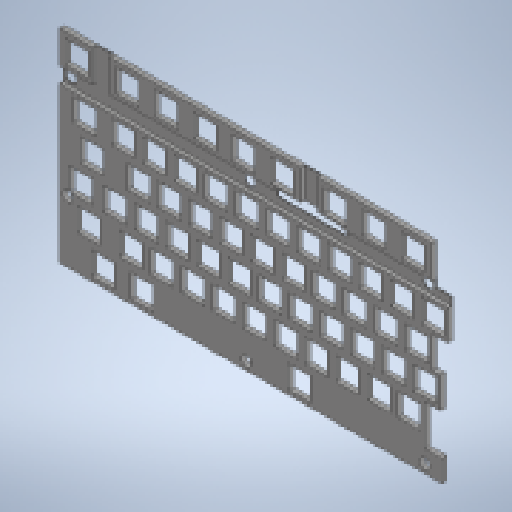
# Autodesk Inventor part: Left Plate
Saved by Autodesk Inventor 2025 (Build 290162000, 162)
## iProperties
Created: 2024-08-12
Part Number: Left Plate
Material: PET Plastic
Document SubType Name: Modeling
Designer: adam
Density: 1.541 g/cm^3
Appearance: Smooth - Medium Gray
Author: adam
Autodesk Inventor part; units mm, degrees
(part 1 of 2)
ref_plane "YZ Plane" through (0, 0, 0) normal (1, 0, 0) x (0, 1, 0)
ref_plane "XZ Plane" through (0, 0, 0) normal (0, 1, 0) x (-1, 0, 0)
ref_plane "XY Plane" through (0, 0, 0) normal (0, 0, 1) x (1, 0, 0)
sketch "Sketch1" plane through (0, 0, 0) normal (0, 0, 1) x (1, 0, 0)
  line L0 (490, -165) -> (40, -165) construction
  line L1 (490, -40) -> (490, -165) construction
  line L2 (40, -40) -> (490, -40) construction
  line L3 (40, -165) -> (40, -40) construction
  circle A0 centre (62.4608, -160.0704) radius 0.725 construction
  circle A1 centre (69.4608, -161.1204) radius 0.725 construction
  circle A2 centre (66.8608, -155.3704) radius 2.55 construction
  circle A3 centre (86.3368, -160.0704) radius 0.725 construction
  circle A4 centre (93.3368, -161.1204) radius 0.725 construction
  circle A5 centre (90.7368, -155.3704) radius 2.55 construction
  line L4 (118.171, -160.2954) -> (124.171, -160.2954) construction
  line L5 (118.171, -145.2954) -> (118.171, -160.2954) construction
  line L6 (124.171, -145.2954) -> (118.171, -145.2954) construction
  line L7 (124.171, -160.2954) -> (124.171, -145.2954) construction
  circle A6 centre (53.5708, -141.0204) radius 0.725 construction
  circle A7 centre (60.5708, -142.0704) radius 0.725 construction
  circle A8 centre (79.7328, -141.0204) radius 0.725 construction
  circle A9 centre (86.7328, -142.0704) radius 0.725 construction
  circle A10 centre (57.9708, -136.3204) radius 2.55 construction
  circle A11 centre (84.1328, -136.3204) radius 2.55 construction
  circle A12 centre (105.7828, -142.0704) radius 0.725 construction
  circle A13 centre (98.7828, -141.0204) radius 0.725 construction
  circle A14 centre (124.8328, -142.0704) radius 0.725 construction
  circle A15 centre (117.8328, -141.0204) radius 0.725 construction
  circle A16 centre (136.8828, -141.0204) radius 0.725 construction
  circle A17 centre (143.8828, -142.0704) radius 0.725 construction
  circle A18 centre (103.1828, -136.3204) radius 2.55 construction
  circle A19 centre (122.2328, -136.3204) radius 2.55 construction
  circle A20 centre (141.2828, -136.3204) radius 2.55 construction
  circle A21 centre (155, -160) radius 1.75 construction
  circle A22 centre (183.5211, -159.9954) radius 0.725 construction
  circle A23 centre (190.5211, -161.0454) radius 0.725 construction
  circle A24 centre (187.9211, -155.2954) radius 2.55 construction
  line L8 (251.6711, -160.2954) -> (257.6711, -160.2954) construction
  line L9 (251.6711, -145.2954) -> (251.6711, -160.2954) construction
  line L10 (257.6711, -145.2954) -> (251.6711, -145.2954) construction
  line L11 (257.6711, -160.2954) -> (257.6711, -145.2954) construction
  circle A25 centre (162.9328, -142.0704) radius 0.725 construction
  circle A26 centre (155.9328, -141.0204) radius 0.725 construction
  circle A27 centre (174.9828, -141.0204) radius 0.725 construction
  circle A28 centre (198, -145.5) radius 0.25 construction
  circle A29 centre (197, -144.5) radius 0.25 construction
  circle A30 centre (181.9828, -142.0704) radius 0.725 construction
  circle A31 centre (194.0328, -141.0204) radius 0.725 construction
  circle A32 centre (201.0328, -142.0704) radius 0.725 construction
  circle A33 centre (160.3328, -136.3204) radius 2.55 construction
  circle A34 centre (179.3828, -136.3204) radius 2.55 construction
  circle A35 centre (166.0148, -132.5036) radius 0.25 construction
  circle A36 centre (198.4328, -136.3204) radius 2.55 construction
  circle A37 centre (210, -146) radius 0.25 construction
  circle A38 centre (220.0828, -142.0704) radius 0.725 construction
  circle A39 centre (213.0828, -141.0204) radius 0.725 construction
  circle A40 centre (232.1368, -141.0224) radius 0.725 construction
  circle A41 centre (239.1368, -142.0724) radius 0.725 construction
  circle A42 centre (258.1768, -142.0924) radius 0.725 construction
  circle A43 centre (251.1768, -141.0424) radius 0.725 construction
  circle A44 centre (217.4828, -136.3204) radius 2.55 construction
  circle A45 centre (236.5368, -136.3224) radius 2.55 construction
  circle A46 centre (255.5768, -136.3424) radius 2.55 construction
  circle A47 centre (45, -127) radius 1.75 construction
  circle A48 centre (55.7448, -123.0204) radius 0.725 construction
  circle A49 centre (48.7448, -121.9704) radius 0.725 construction
  circle A50 centre (70.0808, -121.9704) radius 0.725 construction
  circle A51 centre (53.1448, -117.2704) radius 2.55 construction
  circle A52 centre (77.0808, -123.0204) radius 0.725 construction
  circle A53 centre (96.1308, -123.0204) radius 0.725 construction
  circle A54 centre (89.1308, -121.9704) radius 0.725 construction
  circle A55 centre (74.4808, -117.2704) radius 2.55 construction
  circle A56 centre (93.5308, -117.2704) radius 2.55 construction
  circle A57 centre (108.1808, -121.9704) radius 0.725 construction
  circle A58 centre (115.1808, -123.0204) radius 0.725 construction
  circle A59 centre (112.5808, -117.2704) radius 2.55 construction
  circle A60 centre (134.2308, -123.0204) radius 0.725 construction
  circle A61 centre (127.2308, -121.9704) radius 0.725 construction
  circle A62 centre (153.2808, -123.0204) radius 0.725 construction
  circle A63 centre (146.2808, -121.9704) radius 0.725 construction
  circle A64 centre (131.6308, -117.2704) radius 2.55 construction
  circle A65 centre (150.6808, -117.2704) radius 2.55 construction
  circle A66 centre (68.0148, -110.5036) radius 0.15 construction
  circle A67 centre (75.0148, -110.5036) radius 0.15 construction
  circle A68 centre (55.8568, -102.9204) radius 0.725 construction
  circle A69 centre (62.8568, -103.9704) radius 0.725 construction
  circle A70 centre (85.0148, -106.5036) radius 0.25 construction
  circle A71 centre (84.3048, -102.9204) radius 0.725 construction
  circle A72 centre (91.3048, -103.9704) radius 0.725 construction
  circle A73 centre (142.0148, -113.5036) radius 0.25 construction
  circle A74 centre (123.0148, -107.5036) radius 0.25 construction
  circle A75 centre (110.3548, -103.9704) radius 0.725 construction
  circle A76 centre (103.3548, -102.9204) radius 0.725 construction
  circle A77 centre (122.4048, -102.9204) radius 0.725 construction
  circle A78 centre (129.4048, -103.9704) radius 0.725 construction
  circle A79 centre (148.4548, -103.9704) radius 0.725 construction
  circle A80 centre (141.4548, -102.9204) radius 0.725 construction
  circle A81 centre (165.3308, -121.9704) radius 0.725 construction
  circle A82 centre (172.3308, -123.0204) radius 0.725 construction
  circle A83 centre (169.7308, -117.2704) radius 2.55 construction
  circle A84 centre (191.3808, -123.0204) radius 0.725 construction
  circle A85 centre (184.3808, -121.9704) radius 0.725 construction
  circle A86 centre (203.4308, -121.9704) radius 0.725 construction
  circle A87 centre (188.7808, -117.2704) radius 2.55 construction
  circle A88 centre (207.8308, -117.2704) radius 2.55 construction
  circle A89 centre (223.0148, -125.5036) radius 0.25 construction
  circle A90 centre (210.4308, -123.0204) radius 0.725 construction
  circle A91 centre (222.4808, -121.9704) radius 0.725 construction
  circle A92 centre (229.4808, -123.0204) radius 0.725 construction
  circle A93 centre (226.8808, -117.2704) radius 2.55 construction
  circle A94 centre (248.5308, -123.0204) radius 0.725 construction
  circle A95 centre (241.5308, -121.9704) radius 0.725 construction
  circle A96 centre (260.8348, -121.9704) radius 0.725 construction
  circle A97 centre (245.9308, -117.2704) radius 2.55 construction
  circle A98 centre (167.5048, -104.0492) radius 0.725 construction
  circle A99 centre (160.5048, -102.9992) radius 0.725 construction
  circle A100 centre (179.5548, -102.9204) radius 0.725 construction
  circle A101 centre (199.0148, -108.5036) radius 0.25 construction
  circle A102 centre (186.5548, -103.9704) radius 0.725 construction
  circle A103 centre (205.6048, -103.9704) radius 0.725 construction
  circle A104 centre (198.6048, -102.9204) radius 0.725 construction
  circle A105 centre (217.6548, -102.9204) radius 0.725 construction
  circle A106 centre (224.6548, -103.9704) radius 0.725 construction
  circle A107 centre (236.7048, -102.9204) radius 0.725 construction
  circle A108 centre (243.7048, -103.9704) radius 0.725 construction
  circle A109 centre (262.7548, -103.9704) radius 0.725 construction
  circle A110 centre (255.7548, -102.9204) radius 0.725 construction
  circle A111 centre (265, -160) radius 1.75 construction
  circle A112 centre (281.6628, -160.0704) radius 0.725 construction
  circle A113 centre (288.6628, -161.1204) radius 0.725 construction
  circle A114 centre (280, -155) radius 0.25 construction
  circle A115 centre (286.0628, -155.3704) radius 2.55 construction
  circle A116 centre (305.5388, -160.0704) radius 0.725 construction
  circle A117 centre (312.5388, -161.1204) radius 0.725 construction
  circle A118 centre (302.0148, -157.5036) radius 0.25 construction
  circle A119 centre (309.9388, -155.3704) radius 2.55 construction
  circle A120 centre (305.0148, -151.5036) radius 0.25 construction
  circle A121 centre (304.0148, -150.5036) radius 0.25 construction
  circle A122 centre (375, -160) radius 1.75 construction
  circle A123 centre (277.2328, -142.0704) radius 0.725 construction
  circle A124 centre (270.2328, -141.0204) radius 0.725 construction
  circle A125 centre (306.0468, -141.0204) radius 0.725 construction
  circle A126 centre (313.0468, -142.0704) radius 0.725 construction
  circle A127 centre (274.6328, -136.3204) radius 2.55 construction
  circle A128 centre (278.0148, -132.5036) radius 0.25 construction
  circle A129 centre (310.4468, -136.3204) radius 2.55 construction
  line L12 (295.4468, -141.3204) -> (301.4468, -141.3204) construction
  line L13 (295.4468, -126.3204) -> (295.4468, -141.3204) construction
  line L14 (301.4468, -126.3204) -> (295.4468, -126.3204) construction
  line L15 (301.4468, -141.3204) -> (301.4468, -126.3204) construction
  circle A130 centre (337.0148, -143.5036) radius 0.25 construction
  circle A131 centre (357.43, -142.0196) radius 0.725 construction
  circle A132 centre (350.43, -140.9696) radius 0.725 construction
  circle A133 centre (369.48, -140.9696) radius 0.725 construction
  line L16 (319.4468, -141.3204) -> (325.4468, -141.3204) construction
  line L17 (319.4468, -126.3204) -> (319.4468, -141.3204) construction
  line L18 (325.4468, -126.3204) -> (319.4468, -126.3204) construction
  line L19 (325.4468, -141.3204) -> (325.4468, -126.3204) construction
  circle A134 centre (354.83, -136.2696) radius 2.55 construction
  circle A135 centre (373.88, -136.2696) radius 2.55 construction
  circle A136 centre (426.8108, -159.972) radius 0.725 construction
  circle A137 centre (431.2108, -155.272) radius 2.55 construction
  line L20 (416.2108, -160.272) -> (422.2108, -160.272) construction
  line L21 (416.2108, -145.272) -> (416.2108, -160.272) construction
  line L22 (422.2108, -145.272) -> (416.2108, -145.272) construction
  line L23 (422.2108, -160.272) -> (422.2108, -145.272) construction
  circle A138 centre (433.8108, -161.022) radius 0.725 construction
  circle A139 centre (455.2588, -159.972) radius 0.725 construction
  circle A140 centre (462.2588, -161.022) radius 0.725 construction
  circle A141 centre (459.6588, -155.272) radius 2.55 construction
  line L24 (468.7088, -160.774) -> (483.7088, -160.774) construction
  line L25 (468.7088, -154.774) -> (468.7088, -160.774) construction
  line L26 (483.7088, -154.774) -> (468.7088, -154.774) construction
  line L27 (483.7088, -160.774) -> (483.7088, -154.774) construction
  line L28 (440.2108, -160.272) -> (446.2108, -160.272) construction
  line L29 (440.2108, -145.272) -> (440.2108, -160.272) construction
  line L30 (446.2108, -145.272) -> (440.2108, -145.272) construction
  line L31 (446.2108, -160.272) -> (446.2108, -145.272) construction
  circle A142 centre (455.5, -148.5) radius 0.25 construction
  circle A143 centre (483.4088, -150.174) radius 0.725 construction
  circle A144 centre (376.48, -142.0196) radius 0.725 construction
  circle A145 centre (388.53, -140.9696) radius 0.725 construction
  circle A146 centre (395.53, -142.0196) radius 0.725 construction
  circle A147 centre (412.0148, -145.5036) radius 0.25 construction
  circle A148 centre (417.1588, -140.922) radius 0.725 construction
  circle A149 centre (424.1588, -141.972) radius 0.725 construction
  circle A150 centre (392.93, -136.2696) radius 2.55 construction
  circle A151 centre (421.5588, -136.222) radius 2.55 construction
  circle A152 centre (443.2088, -141.972) radius 0.725 construction
  circle A153 centre (436.2088, -140.922) radius 0.725 construction
  circle A154 centre (455.2588, -140.922) radius 0.725 construction
  circle A155 centre (478.7088, -145.774) radius 2.55 construction
  circle A156 centre (484.4588, -143.174) radius 0.725 construction
  circle A157 centre (462.2588, -141.972) radius 0.725 construction
  circle A158 centre (440.6088, -136.222) radius 2.55 construction
  circle A159 centre (459.6588, -136.222) radius 2.55 construction
  line L32 (468.7088, -136.774) -> (483.7088, -136.774) construction
  line L33 (468.7088, -130.774) -> (468.7088, -136.774) construction
  line L34 (483.7088, -130.774) -> (468.7088, -130.774) construction
  line L35 (483.7088, -136.774) -> (483.7088, -130.774) construction
  circle A160 centre (303, -126.5) radius 0.25 construction
  circle A161 centre (309.0148, -126.5036) radius 0.25 construction
  circle A162 centre (267.8348, -123.0204) radius 0.725 construction
  circle A163 centre (286.8848, -123.0204) radius 0.725 construction
  circle A164 centre (279.8848, -121.9704) radius 0.725 construction
  circle A165 centre (265.2348, -117.2704) radius 2.55 construction
  circle A166 centre (284.2848, -117.2704) radius 2.55 construction
  circle A167 centre (305.9348, -123.0204) radius 0.725 construction
  circle A168 centre (298.9348, -121.9704) radius 0.725 construction
  circle A169 centre (303.3348, -117.2704) radius 2.55 construction
  circle A170 centre (362.0148, -127.5036) radius 0.25 construction
  line L36 (315.6708, -122.8724) -> (330.6708, -122.8724) construction
  line L37 (315.6708, -116.8724) -> (315.6708, -122.8724) construction
  line L38 (330.6708, -116.8724) -> (315.6708, -116.8724) construction
  line L39 (330.6708, -122.8724) -> (330.6708, -116.8724) construction
  circle A171 centre (369.48, -121.9196) radius 0.725 construction
  circle A172 centre (373.88, -117.2196) radius 2.55 construction
  circle A173 centre (275.0148, -112.5036) radius 0.25 construction
  circle A174 centre (310.0148, -116.5036) radius 0.25 construction
  circle A175 centre (274.8048, -102.9204) radius 0.725 construction
  circle A176 centre (281.8048, -103.9704) radius 0.725 construction
  circle A177 centre (300.8548, -103.9704) radius 0.725 construction
  circle A178 centre (293.8548, -102.9204) radius 0.725 construction
  circle A179 centre (329.3458, -112.2974) radius 0.725 construction
  circle A180 centre (324.6458, -107.8974) radius 2.55 construction
  circle A181 centre (330.3958, -105.2974) radius 0.725 construction
  circle A182 centre (335.0148, -102.5036) radius 0.25 construction
  circle A183 centre (358.0148, -102.5036) radius 0.25 construction
  circle A184 centre (376.48, -122.9696) radius 0.725 construction
  circle A185 centre (417.1588, -121.872) radius 0.725 construction
  circle A186 centre (424.1588, -122.922) radius 0.725 construction
  circle A187 centre (421.5588, -117.172) radius 2.55 construction
  circle A188 centre (485, -127) radius 1.75 construction
  circle A189 centre (443.2088, -122.922) radius 0.725 construction
  circle A190 centre (436.2088, -121.872) radius 0.725 construction
  circle A191 centre (455.2588, -121.872) radius 0.725 construction
  circle A192 centre (440.6088, -117.172) radius 2.55 construction
  circle A193 centre (462.2588, -122.922) radius 0.725 construction
  circle A194 centre (481.3088, -122.922) radius 0.725 construction
  circle A195 centre (474.3088, -121.872) radius 0.725 construction
  circle A196 centre (459.6588, -117.172) radius 2.55 construction
  circle A197 centre (478.7088, -117.172) radius 2.55 construction
  circle A198 centre (411.0148, -106.5036) radius 0.25 construction
  circle A199 centre (417.1588, -102.822) radius 0.725 construction
  circle A200 centre (424.1588, -103.872) radius 0.725 construction
  circle A201 centre (436.2088, -102.822) radius 0.725 construction
  circle A202 centre (443.2088, -103.872) radius 0.725 construction
  circle A203 centre (455.2588, -102.822) radius 0.725 construction
  circle A204 centre (462.2588, -103.872) radius 0.725 construction
  circle A205 centre (474.3088, -102.822) radius 0.725 construction
  circle A206 centre (481.3088, -103.872) radius 0.725 construction
  line L40 (45.2568, -103.2204) -> (51.2568, -103.2204) construction
  line L41 (45.2568, -88.2204) -> (45.2568, -103.2204) construction
  line L42 (51.2568, -88.2204) -> (45.2568, -88.2204) construction
  line L43 (51.2568, -103.2204) -> (51.2568, -88.2204) construction
  circle A207 centre (60.2568, -98.2204) radius 2.55 construction
  line L44 (69.2568, -103.2204) -> (75.2568, -103.2204) construction
  line L45 (69.2568, -88.2204) -> (69.2568, -103.2204) construction
  line L46 (75.2568, -88.2204) -> (69.2568, -88.2204) construction
  line L47 (75.2568, -103.2204) -> (75.2568, -88.2204) construction
  circle A208 centre (88.7048, -98.2204) radius 2.55 construction
  circle A209 centre (94.0148, -90.5036) radius 0.25 construction
  circle A210 centre (107.7548, -98.2204) radius 2.55 construction
  circle A211 centre (126.8048, -98.2204) radius 2.55 construction
  circle A212 centre (145.8548, -98.2204) radius 2.55 construction
  circle A213 centre (51.1288, -83.8704) radius 0.725 construction
  circle A214 centre (58.1288, -84.9204) radius 0.725 construction
  circle A215 centre (74.9068, -83.8704) radius 0.725 construction
  circle A216 centre (81.9068, -84.9204) radius 0.725 construction
  circle A217 centre (93.9568, -83.8704) radius 0.725 construction
  circle A218 centre (55.5288, -79.1704) radius 2.55 construction
  circle A219 centre (50, -75) radius 0.25 construction
  circle A220 centre (79.3068, -79.1704) radius 2.55 construction
  circle A221 centre (98.3568, -79.1704) radius 2.55 construction
  circle A222 centre (100.9568, -84.9204) radius 0.725 construction
  circle A223 centre (113.0068, -83.8704) radius 0.725 construction
  circle A224 centre (120.0068, -84.9204) radius 0.725 construction
  circle A225 centre (132.0568, -83.8704) radius 0.725 construction
  circle A226 centre (139.0568, -84.9204) radius 0.725 construction
  circle A227 centre (151.1068, -83.8704) radius 0.725 construction
  circle A228 centre (117.4068, -79.1704) radius 2.55 construction
  circle A229 centre (110.5, -73) radius 0.25 construction
  circle A230 centre (136.4568, -79.1704) radius 2.55 construction
  circle A231 centre (164.9048, -98.2992) radius 2.55 construction
  circle A232 centre (183.9548, -98.2204) radius 2.55 construction
  circle A233 centre (203.0048, -98.2204) radius 2.55 construction
  circle A234 centre (177.0148, -92.5036) radius 0.25 construction
  circle A235 centre (176.0148, -91.5036) radius 0.25 construction
  circle A236 centre (200.0148, -91.5036) radius 0.25 construction
  circle A237 centre (192.0148, -89.5036) radius 0.25 construction
  circle A238 centre (199.0148, -90.5036) radius 0.25 construction
  circle A239 centre (222.0548, -98.2204) radius 2.55 construction
  circle A240 centre (241.1048, -98.2204) radius 2.55 construction
  circle A241 centre (260.1548, -98.2204) radius 2.55 construction
  circle A242 centre (247.0148, -93.5036) radius 0.25 construction
  circle A243 centre (158.1068, -84.9204) radius 0.725 construction
  circle A244 centre (170.1568, -83.8704) radius 0.725 construction
  circle A245 centre (177.1568, -84.9204) radius 0.725 construction
  circle A246 centre (189.2068, -83.8704) radius 0.725 construction
  circle A247 centre (196.2068, -84.9204) radius 0.725 construction
  circle A248 centre (208.2568, -83.8704) radius 0.725 construction
  circle A249 centre (200.0148, -82.5036) radius 0.25 construction
  circle A250 centre (155.5068, -79.1704) radius 2.55 construction
  circle A251 centre (174.5568, -79.1704) radius 2.55 construction
  circle A252 centre (155.5, -74.5) radius 0.25 construction
  circle A253 centre (193.6068, -79.1704) radius 2.55 construction
  circle A254 centre (215.2568, -84.9204) radius 0.725 construction
  circle A255 centre (227.3068, -83.8704) radius 0.725 construction
  circle A256 centre (234.3068, -84.9204) radius 0.725 construction
  circle A257 centre (246.3568, -83.8704) radius 0.725 construction
  circle A258 centre (253.3568, -84.9204) radius 0.725 construction
  circle A259 centre (212.6568, -79.1704) radius 2.55 construction
  circle A260 centre (231.7068, -79.1704) radius 2.55 construction
  circle A261 centre (228.0148, -74.5036) radius 0.25 construction
  circle A262 centre (250.7568, -79.1704) radius 2.55 construction
  circle A263 centre (45, -64.8616) radius 1.75 construction
  circle A264 centre (75, -71.5) radius 0.25 construction
  circle A265 centre (49.5, -62) radius 0.25 construction
  circle A266 centre (68.0148, -60.5036) radius 0.25 construction
  circle A267 centre (74.5148, -58.0036) radius 0.25 construction
  circle A268 centre (50, -56.0036) radius 0.25 construction
  circle A269 centre (48, -55) radius 0.25 construction
  circle A270 centre (50.8588, -50.6116) radius 2.55 construction
  circle A271 centre (81.9072, -50.3984) radius 2.55 construction
  circle A272 centre (48.2588, -44.8616) radius 0.725 construction
  circle A273 centre (55.2588, -45.9116) radius 0.725 construction
  circle A274 centre (79.3072, -44.6484) radius 0.725 construction
  circle A275 centre (86.3072, -45.6984) radius 0.725 construction
  circle A276 centre (105.7228, -50.5136) radius 2.55 construction
  circle A277 centre (134.0148, -57.0036) radius 0.25 construction
  circle A278 centre (129.5988, -50.5416) radius 2.55 construction
  circle A279 centre (153.4748, -50.5136) radius 2.55 construction
  circle A280 centre (103.1228, -44.7636) radius 0.725 construction
  circle A281 centre (110.1228, -45.8136) radius 0.725 construction
  circle A282 centre (126.9988, -44.7916) radius 0.725 construction
  circle A283 centre (133.9988, -45.8416) radius 0.725 construction
  circle A284 centre (150.8748, -44.7636) radius 0.725 construction
  circle A285 centre (155, -64.8616) radius 1.75 construction
  circle A286 centre (175.2648, -63.1601) radius 0.425 construction
  circle A287 centre (177.7648, -63.1601) radius 0.425 construction
  circle A288 centre (180.2648, -63.1601) radius 0.425 construction
  circle A289 centre (174.0148, -60.6601) radius 0.425 construction
  circle A290 centre (176.5148, -60.6601) radius 0.425 construction
  circle A291 centre (179.0148, -60.6601) radius 0.425 construction
  circle A292 centre (181.5148, -60.6601) radius 0.425 construction
  circle A293 centre (182.7648, -63.1601) radius 0.425 construction
  circle A294 centre (185.2648, -63.1601) radius 0.425 construction
  circle A295 centre (187.7648, -63.1601) radius 0.425 construction
  circle A296 centre (190.2648, -63.1601) radius 0.425 construction
  circle A297 centre (192.7648, -63.1601) radius 0.425 construction
  circle A298 centre (195.2648, -63.1601) radius 0.425 construction
  circle A299 centre (197.7648, -63.1601) radius 0.425 construction
  circle A300 centre (200.2648, -63.1601) radius 0.425 construction
  circle A301 centre (202.7648, -63.1601) radius 0.425 construction
  circle A302 centre (205.2648, -63.1601) radius 0.425 construction
  circle A303 centre (207.7648, -63.1601) radius 0.425 construction
  circle A304 centre (184.0148, -60.6601) radius 0.425 construction
  circle A305 centre (186.5148, -60.6601) radius 0.425 construction
  circle A306 centre (189.0148, -60.6601) radius 0.425 construction
  circle A307 centre (191.5148, -60.6601) radius 0.425 construction
  circle A308 centre (194.0148, -60.6601) radius 0.425 construction
  circle A309 centre (196.5148, -60.6601) radius 0.425 construction
  circle A310 centre (199.0148, -60.6601) radius 0.425 construction
  circle A311 centre (201.5148, -60.6601) radius 0.425 construction
  circle A312 centre (204.0148, -60.6601) radius 0.425 construction
  circle A313 centre (206.5148, -60.6601) radius 0.425 construction
  circle A314 centre (209.0148, -60.6601) radius 0.425 construction
  circle A315 centre (228.0148, -68.5036) radius 0.25 construction
  circle A316 centre (259.5, -67.5036) radius 0.25 construction
  circle A317 centre (210.2648, -63.1601) radius 0.425 construction
  circle A318 centre (212.7648, -63.1601) radius 0.425 construction
  circle A319 centre (211.5148, -60.6601) radius 0.425 construction
  circle A320 centre (211.5148, -58.0036) radius 0.25 construction
  circle A321 centre (177.3508, -50.5136) radius 2.55 construction
  circle A322 centre (189.0148, -56.0036) radius 0.25 construction
  circle A323 centre (186.5148, -55.0036) radius 0.25 construction
  circle A324 centre (196.5148, -57.0036) radius 0.25 construction
  circle A325 centre (204.0148, -54.5036) radius 0.25 construction
  circle A326 centre (157.8748, -45.8136) radius 0.725 construction
  circle A327 centre (174.7508, -44.7636) radius 0.725 construction
  circle A328 centre (181.7508, -45.8136) radius 0.725 construction
  circle A329 centre (202.0148, -47.5036) radius 0.25 construction
  circle A330 centre (199.0148, -46.5036) radius 0.25 construction
  circle A331 centre (207.2568, -44.7636) radius 0.725 construction
  circle A332 centre (209.8568, -50.5136) radius 2.55 construction
  circle A333 centre (233.7388, -50.5136) radius 2.55 construction
  circle A334 centre (257.6148, -50.5136) radius 2.55 construction
  circle A335 centre (214.2568, -45.8136) radius 0.725 construction
  circle A336 centre (231.1388, -44.7636) radius 0.725 construction
  circle A337 centre (238.1388, -45.8136) radius 0.725 construction
  circle A338 centre (255.0148, -44.7636) radius 0.725 construction
  circle A339 centre (262.0148, -45.8136) radius 0.725 construction
  circle A340 centre (279.2048, -98.2204) radius 2.55 construction
  circle A341 centre (298.2548, -98.2204) radius 2.55 construction
  circle A342 centre (301.0148, -87.5036) radius 0.25 construction
  circle A343 centre (313.0148, -87.5036) radius 0.25 construction
  line L48 (315.6708, -98.8724) -> (330.6708, -98.8724) construction
  line L49 (315.6708, -92.8724) -> (315.6708, -98.8724) construction
  line L50 (330.6708, -92.8724) -> (315.6708, -92.8724) construction
  line L51 (330.6708, -98.8724) -> (330.6708, -92.8724) construction
  circle A344 centre (265.4068, -83.8704) radius 0.725 construction
  circle A345 centre (272.4068, -84.9204) radius 0.725 construction
  circle A346 centre (284.4568, -83.8704) radius 0.725 construction
  circle A347 centre (291.4568, -84.9204) radius 0.725 construction
  circle A348 centre (303.5068, -83.8704) radius 0.725 construction
  circle A349 centre (310.5068, -84.9204) radius 0.725 construction
  circle A350 centre (269.8068, -79.1704) radius 2.55 construction
  circle A351 centre (288.8568, -79.1704) radius 2.55 construction
  circle A352 centre (307.9068, -79.1704) radius 2.55 construction
  circle A353 centre (322.5568, -83.8704) radius 0.725 construction
  circle A354 centre (329.5568, -84.9204) radius 0.725 construction
  circle A355 centre (355.158, -83.8056) radius 0.725 construction
  circle A356 centre (362.158, -84.8556) radius 0.725 construction
  circle A357 centre (326.9568, -79.1704) radius 2.55 construction
  circle A358 centre (359.558, -79.1056) radius 2.55 construction
  circle A359 centre (421.5588, -98.122) radius 2.55 construction
  circle A360 centre (384.0148, -89.5036) radius 0.25 construction
  circle A361 centre (440.6088, -98.122) radius 2.55 construction
  circle A362 centre (459.6588, -98.122) radius 2.55 construction
  circle A363 centre (478.7088, -98.122) radius 2.55 construction
  circle A364 centre (383.754, -83.8056) radius 0.725 construction
  circle A365 centre (390.754, -84.8556) radius 0.725 construction
  circle A366 centre (411.0148, -83.5036) radius 0.25 construction
  circle A367 centre (417.1588, -83.772) radius 0.725 construction
  circle A368 centre (424.1588, -84.822) radius 0.725 construction
  circle A369 centre (412.0148, -82.5036) radius 0.25 construction
  circle A370 centre (388.154, -79.1056) radius 2.55 construction
  circle A371 centre (421.5588, -79.072) radius 2.55 construction
  circle A372 centre (436.2088, -83.772) radius 0.725 construction
  circle A373 centre (443.2088, -84.822) radius 0.725 construction
  circle A374 centre (455.2588, -83.772) radius 0.725 construction
  circle A375 centre (462.2588, -84.822) radius 0.725 construction
  circle A376 centre (474.3088, -83.772) radius 0.725 construction
  circle A377 centre (481.3088, -84.822) radius 0.725 construction
  circle A378 centre (440.6088, -79.072) radius 2.55 construction
  circle A379 centre (459.6588, -79.072) radius 2.55 construction
  circle A380 centre (478.7088, -79.072) radius 2.55 construction
  circle A381 centre (265, -64.8616) radius 1.75 construction
  circle A382 centre (303.5, -69) radius 0.25 construction
  circle A383 centre (286, -59) radius 0.25 construction
  circle A384 centre (314.5, -61) radius 0.25 construction
  circle A385 centre (311, -60) radius 0.25 construction
  circle A386 centre (375, -64.8616) radius 1.75 construction
  circle A387 centre (281.4908, -50.5136) radius 2.55 construction
  circle A388 centre (305.3668, -50.5136) radius 2.55 construction
  circle A389 centre (278.8908, -44.7636) radius 0.725 construction
  circle A390 centre (285.8908, -45.8136) radius 0.725 construction
  circle A391 centre (302.7668, -44.7636) radius 0.725 construction
  circle A392 centre (309.7668, -45.8136) radius 0.725 construction
  circle A393 centre (333.3668, -48.0136) radius 5 construction
  circle A394 centre (485, -64.8616) radius 1.75 construction
  circle A395 centre (463, -60.5) radius 0.25 construction
  circle A396 centre (408.3668, -48.0136) radius 5 construction
  circle A397 centre (453.2088, -50.322) radius 5 construction
  circle A398 centre (466.5, -56.5) radius 0.25 construction
  circle A399 centre (481.2088, -50.322) radius 5 construction
  circle A400 centre (447, -47) radius 0.25 construction
  circle A401 centre (432.68, -43) radius 0.5 construction
  circle A402 centre (435.22, -43) radius 0.5 construction
  circle A403 centre (437.76, -43) radius 0.5 construction
  circle A404 centre (440.3, -43) radius 0.5 construction
  circle A405 centre (460.5, -42.5) radius 0.25 construction
  circle A406 centre (468, -44) radius 0.25 construction
  circle A407 centre (155, -160) radius 3.25
  circle A408 centre (265, -160) radius 3.25
  line L52 (43.8563, -57.6141) -> (57.8613, -57.6141)
  line L53 (57.8613, -57.6141) -> (57.8613, -43.6091)
  line L54 (57.8613, -43.6091) -> (43.8563, -43.6091)
  line L55 (43.8563, -43.6091) -> (43.8563, -57.6141)
  line L56 (43.8563, -57.6141) -> (57.8613, -43.6091) construction
  line L57 (57.8613, -57.6141) -> (43.8563, -43.6091) construction
  line L58 (74.9047, -43.3959) -> (88.9097, -43.3959)
  line L59 (88.9097, -43.3959) -> (88.9097, -57.4009)
  line L60 (88.9097, -57.4009) -> (74.9047, -57.4009)
  line L61 (74.9047, -57.4009) -> (74.9047, -43.3959)
  line L62 (74.9047, -43.3959) -> (88.9097, -57.4009) construction
  line L63 (88.9097, -43.3959) -> (74.9047, -57.4009) construction
  line L64 (98.7203, -43.5111) -> (112.7253, -43.5111)
  line L65 (112.7253, -43.5111) -> (112.7253, -57.5161)
  line L66 (112.7253, -57.5161) -> (98.7203, -57.5161)
  line L67 (98.7203, -57.5161) -> (98.7203, -43.5111)
  line L68 (98.7203, -43.5111) -> (112.7253, -57.5161) construction
  line L69 (112.7253, -43.5111) -> (98.7203, -57.5161) construction
  line L70 (122.5963, -43.5391) -> (136.6013, -43.5391)
  line L71 (136.6013, -43.5391) -> (136.6013, -57.5441)
  line L72 (136.6013, -57.5441) -> (122.5963, -57.5441)
  line L73 (122.5963, -57.5441) -> (122.5963, -43.5391)
  line L74 (122.5963, -43.5391) -> (136.6013, -57.5441) construction
  line L75 (136.6013, -43.5391) -> (122.5963, -57.5441) construction
  line L76 (146.4723, -43.5111) -> (160.4773, -43.5111)
  line L77 (160.4773, -43.5111) -> (160.4773, -57.5161)
  line L78 (160.4773, -57.5161) -> (146.4723, -57.5161)
  line L79 (146.4723, -57.5161) -> (146.4723, -43.5111)
  line L80 (146.4723, -43.5111) -> (160.4773, -57.5161) construction
  line L81 (160.4773, -43.5111) -> (146.4723, -57.5161) construction
  line L82 (170.3483, -43.5111) -> (184.3533, -43.5111)
  line L83 (184.3533, -43.5111) -> (184.3533, -57.5161)
  line L84 (184.3533, -57.5161) -> (170.3483, -57.5161)
  line L85 (170.3483, -57.5161) -> (170.3483, -43.5111)
  line L86 (170.3483, -43.5111) -> (184.3533, -57.5161) construction
  line L87 (184.3533, -43.5111) -> (170.3483, -57.5161) construction
  line L88 (202.8543, -43.5111) -> (216.8593, -43.5111)
  line L89 (216.8593, -43.5111) -> (216.8593, -57.5161)
  line L90 (216.8593, -57.5161) -> (202.8543, -57.5161)
  line L91 (202.8543, -57.5161) -> (202.8543, -43.5111)
  line L92 (202.8543, -43.5111) -> (216.8593, -57.5161) construction
  line L93 (216.8593, -43.5111) -> (202.8543, -57.5161) construction
  line L94 (226.7363, -43.5111) -> (240.7413, -43.5111)
  line L95 (240.7413, -43.5111) -> (240.7413, -57.5161)
  line L96 (240.7413, -57.5161) -> (226.7363, -57.5161)
  line L97 (226.7363, -57.5161) -> (226.7363, -43.5111)
  line L98 (226.7363, -43.5111) -> (240.7413, -57.5161) construction
  line L99 (240.7413, -43.5111) -> (226.7363, -57.5161) construction
  line L100 (250.6123, -43.5111) -> (264.6173, -43.5111)
  line L101 (264.6173, -43.5111) -> (264.6173, -57.5161)
  line L102 (264.6173, -57.5161) -> (250.6123, -57.5161)
  line L103 (250.6123, -57.5161) -> (250.6123, -43.5111)
  line L104 (250.6123, -43.5111) -> (264.6173, -57.5161) construction
  line L105 (264.6173, -43.5111) -> (250.6123, -57.5161) construction
  line L106 (262.8043, -72.1679) -> (276.8093, -72.1679)
  line L107 (276.8093, -72.1679) -> (276.8093, -86.1729)
  line L108 (276.8093, -86.1729) -> (262.8043, -86.1729)
  line L109 (262.8043, -86.1729) -> (262.8043, -72.1679)
  line L110 (262.8043, -72.1679) -> (276.8093, -86.1729) construction
  line L111 (276.8093, -72.1679) -> (262.8043, -86.1729) construction
  line L112 (253.1523, -91.2179) -> (267.1573, -91.2179)
  line L113 (267.1573, -91.2179) -> (267.1573, -105.2229)
  line L114 (267.1573, -105.2229) -> (253.1523, -105.2229)
  line L115 (253.1523, -105.2229) -> (253.1523, -91.2179)
  line L116 (253.1523, -91.2179) -> (267.1573, -105.2229) construction
  line L117 (267.1573, -91.2179) -> (253.1523, -105.2229) construction
  line L118 (258.2323, -110.2679) -> (272.2373, -110.2679)
  line L119 (272.2373, -110.2679) -> (272.2373, -124.2729)
  line L120 (272.2373, -124.2729) -> (258.2323, -124.2729)
  line L121 (258.2323, -124.2729) -> (258.2323, -110.2679)
  line L122 (258.2323, -110.2679) -> (272.2373, -124.2729) construction
  line L123 (272.2373, -110.2679) -> (258.2323, -124.2729) construction
  line L124 (248.5743, -129.3399) -> (262.5793, -129.3399)
  line L125 (262.5793, -129.3399) -> (262.5793, -143.3449)
  line L126 (262.5793, -143.3449) -> (248.5743, -143.3449)
  line L127 (248.5743, -143.3449) -> (248.5743, -129.3399)
  line L128 (248.5743, -129.3399) -> (262.5793, -143.3449) construction
  line L129 (262.5793, -129.3399) -> (248.5743, -143.3449) construction
  line L130 (229.5343, -129.3199) -> (243.5393, -129.3199)
  line L131 (243.5393, -129.3199) -> (243.5393, -143.3249)
  line L132 (243.5393, -143.3249) -> (229.5343, -143.3249)
  line L133 (229.5343, -143.3249) -> (229.5343, -129.3199)
  line L134 (229.5343, -129.3199) -> (243.5393, -143.3249) construction
  line L135 (243.5393, -129.3199) -> (229.5343, -143.3249) construction
  line L136 (238.9283, -110.2679) -> (252.9333, -110.2679)
  line L137 (252.9333, -110.2679) -> (252.9333, -124.2729)
  line L138 (252.9333, -124.2729) -> (238.9283, -124.2729)
  line L139 (238.9283, -124.2729) -> (238.9283, -110.2679)
  line L140 (238.9283, -110.2679) -> (252.9333, -124.2729) construction
  line L141 (252.9333, -110.2679) -> (238.9283, -124.2729) construction
  line L142 (234.1023, -91.2179) -> (248.1073, -91.2179)
  line L143 (248.1073, -91.2179) -> (248.1073, -105.2229)
  line L144 (248.1073, -105.2229) -> (234.1023, -105.2229)
  line L145 (234.1023, -105.2229) -> (234.1023, -91.2179)
  line L146 (234.1023, -91.2179) -> (248.1073, -105.2229) construction
  line L147 (248.1073, -91.2179) -> (234.1023, -105.2229) construction
  line L148 (243.7543, -72.1679) -> (257.7593, -72.1679)
  line L149 (257.7593, -72.1679) -> (257.7593, -86.1729)
  line L150 (257.7593, -86.1729) -> (243.7543, -86.1729)
  line L151 (243.7543, -86.1729) -> (243.7543, -72.1679)
  line L152 (243.7543, -72.1679) -> (257.7593, -86.1729) construction
  line L153 (257.7593, -72.1679) -> (243.7543, -86.1729) construction
  line L154 (224.7043, -72.1679) -> (238.7093, -72.1679)
  line L155 (238.7093, -72.1679) -> (238.7093, -86.1729)
  line L156 (238.7093, -86.1729) -> (224.7043, -86.1729)
  line L157 (224.7043, -86.1729) -> (224.7043, -72.1679)
  line L158 (224.7043, -72.1679) -> (238.7093, -86.1729) construction
  line L159 (238.7093, -72.1679) -> (224.7043, -86.1729) construction
  line L160 (205.6543, -72.1679) -> (219.6593, -72.1679)
  line L161 (219.6593, -72.1679) -> (219.6593, -86.1729)
  line L162 (219.6593, -86.1729) -> (205.6543, -86.1729)
  line L163 (205.6543, -86.1729) -> (205.6543, -72.1679)
  line L164 (205.6543, -72.1679) -> (219.6593, -86.1729) construction
  line L165 (219.6593, -72.1679) -> (205.6543, -86.1729) construction
  line L166 (186.6043, -72.1679) -> (200.6093, -72.1679)
  line L167 (200.6093, -72.1679) -> (200.6093, -86.1729)
  line L168 (200.6093, -86.1729) -> (186.6043, -86.1729)
  line L169 (186.6043, -86.1729) -> (186.6043, -72.1679)
  line L170 (186.6043, -72.1679) -> (200.6093, -86.1729) construction
  line L171 (200.6093, -72.1679) -> (186.6043, -86.1729) construction
  line L172 (167.5543, -72.1679) -> (181.5593, -72.1679)
  line L173 (181.5593, -72.1679) -> (181.5593, -86.1729)
  line L174 (181.5593, -86.1729) -> (167.5543, -86.1729)
  line L175 (167.5543, -86.1729) -> (167.5543, -72.1679)
  line L176 (167.5543, -72.1679) -> (181.5593, -86.1729) construction
  line L177 (181.5593, -72.1679) -> (167.5543, -86.1729) construction
  line L178 (148.5043, -72.1679) -> (162.5093, -72.1679)
  line L179 (162.5093, -72.1679) -> (162.5093, -86.1729)
  line L180 (162.5093, -86.1729) -> (148.5043, -86.1729)
  line L181 (148.5043, -86.1729) -> (148.5043, -72.1679)
  line L182 (148.5043, -72.1679) -> (162.5093, -86.1729) construction
  line L183 (162.5093, -72.1679) -> (148.5043, -86.1729) construction
  line L184 (129.4543, -72.1679) -> (143.4593, -72.1679)
  line L185 (143.4593, -72.1679) -> (143.4593, -86.1729)
  line L186 (143.4593, -86.1729) -> (129.4543, -86.1729)
  line L187 (129.4543, -86.1729) -> (129.4543, -72.1679)
  line L188 (129.4543, -72.1679) -> (143.4593, -86.1729) construction
  line L189 (143.4593, -72.1679) -> (129.4543, -86.1729) construction
  line L190 (110.4043, -72.1679) -> (124.4093, -72.1679)
  line L191 (124.4093, -72.1679) -> (124.4093, -86.1729)
  line L192 (124.4093, -86.1729) -> (110.4043, -86.1729)
  line L193 (110.4043, -86.1729) -> (110.4043, -72.1679)
  line L194 (110.4043, -72.1679) -> (124.4093, -86.1729) construction
  line L195 (124.4093, -72.1679) -> (110.4043, -86.1729) construction
  line L196 (91.3543, -72.1679) -> (105.3593, -72.1679)
  line L197 (105.3593, -72.1679) -> (105.3593, -86.1729)
  line L198 (105.3593, -86.1729) -> (91.3543, -86.1729)
  line L199 (91.3543, -86.1729) -> (91.3543, -72.1679)
  line L200 (91.3543, -72.1679) -> (105.3593, -86.1729) construction
  line L201 (105.3593, -72.1679) -> (91.3543, -86.1729) construction
  line L202 (72.3043, -72.1679) -> (86.3093, -72.1679)
  line L203 (86.3093, -72.1679) -> (86.3093, -86.1729)
  line L204 (86.3093, -86.1729) -> (72.3043, -86.1729)
  line L205 (72.3043, -86.1729) -> (72.3043, -72.1679)
  line L206 (72.3043, -72.1679) -> (86.3093, -86.1729) construction
  line L207 (86.3093, -72.1679) -> (72.3043, -86.1729) construction
  line L208 (48.5263, -72.1679) -> (62.5313, -72.1679)
  line L209 (62.5313, -72.1679) -> (62.5313, -86.1729)
  line L210 (62.5313, -86.1729) -> (48.5263, -86.1729)
  line L211 (48.5263, -86.1729) -> (48.5263, -72.1679)
  line L212 (48.5263, -72.1679) -> (62.5313, -86.1729) construction
  line L213 (62.5313, -72.1679) -> (48.5263, -86.1729) construction
  line L214 (53.2543, -91.2179) -> (67.2593, -91.2179)
  line L215 (67.2593, -91.2179) -> (67.2593, -105.2229)
  line L216 (67.2593, -105.2229) -> (53.2543, -105.2229)
  line L217 (53.2543, -105.2229) -> (53.2543, -91.2179)
  line L218 (53.2543, -91.2179) -> (67.2593, -105.2229) construction
  line L219 (67.2593, -91.2179) -> (53.2543, -105.2229) construction
  line L220 (81.7023, -91.2179) -> (95.7073, -91.2179)
  line L221 (95.7073, -91.2179) -> (95.7073, -105.2229)
  line L222 (95.7073, -105.2229) -> (81.7023, -105.2229)
  line L223 (81.7023, -105.2229) -> (81.7023, -91.2179)
  line L224 (81.7023, -91.2179) -> (95.7073, -105.2229) construction
  line L225 (95.7073, -91.2179) -> (81.7023, -105.2229) construction
  line L226 (46.1423, -110.2679) -> (60.1473, -110.2679)
  line L227 (60.1473, -110.2679) -> (60.1473, -124.2729)
  line L228 (60.1473, -124.2729) -> (46.1423, -124.2729)
  line L229 (46.1423, -124.2729) -> (46.1423, -110.2679)
  line L230 (46.1423, -110.2679) -> (60.1473, -124.2729) construction
  line L231 (60.1473, -110.2679) -> (46.1423, -124.2729) construction
  line L232 (67.4783, -110.2679) -> (81.4833, -110.2679)
  line L233 (81.4833, -110.2679) -> (81.4833, -124.2729)
  line L234 (81.4833, -124.2729) -> (67.4783, -124.2729)
  line L235 (67.4783, -124.2729) -> (67.4783, -110.2679)
  line L236 (67.4783, -110.2679) -> (81.4833, -124.2729) construction
  line L237 (81.4833, -110.2679) -> (67.4783, -124.2729) construction
  line L238 (50.9683, -129.3179) -> (64.9733, -129.3179)
  line L239 (64.9733, -129.3179) -> (64.9733, -143.3229)
  line L240 (64.9733, -143.3229) -> (50.9683, -143.3229)
  line L241 (50.9683, -143.3229) -> (50.9683, -129.3179)
  line L242 (50.9683, -129.3179) -> (64.9733, -143.3229) construction
  line L243 (64.9733, -129.3179) -> (50.9683, -143.3229) construction
  line L244 (59.8583, -148.3679) -> (73.8633, -148.3679)
  line L245 (73.8633, -148.3679) -> (73.8633, -162.3729)
  line L246 (73.8633, -162.3729) -> (59.8583, -162.3729)
  line L247 (59.8583, -162.3729) -> (59.8583, -148.3679)
  line L248 (59.8583, -148.3679) -> (73.8633, -162.3729) construction
  line L249 (73.8633, -148.3679) -> (59.8583, -162.3729) construction
  line L250 (83.7343, -148.3679) -> (97.7393, -148.3679)
  line L251 (97.7393, -148.3679) -> (97.7393, -162.3729)
  line L252 (97.7393, -162.3729) -> (83.7343, -162.3729)
  line L253 (83.7343, -162.3729) -> (83.7343, -148.3679)
  line L254 (83.7343, -148.3679) -> (97.7393, -162.3729) construction
  line L255 (97.7393, -148.3679) -> (83.7343, -162.3729) construction
  line L256 (77.1303, -129.3179) -> (91.1353, -129.3179)
  line L257 (91.1353, -129.3179) -> (91.1353, -143.3229)
  line L258 (91.1353, -143.3229) -> (77.1303, -143.3229)
  line L259 (77.1303, -143.3229) -> (77.1303, -129.3179)
  line L260 (77.1303, -129.3179) -> (91.1353, -143.3229) construction
  line L261 (91.1353, -129.3179) -> (77.1303, -143.3229) construction
  line L262 (86.5283, -110.2679) -> (100.5333, -110.2679)
  line L263 (100.5333, -110.2679) -> (100.5333, -124.2729)
  line L264 (100.5333, -124.2729) -> (86.5283, -124.2729)
  line L265 (86.5283, -124.2729) -> (86.5283, -110.2679)
  line L266 (86.5283, -110.2679) -> (100.5333, -124.2729) construction
  line L267 (100.5333, -110.2679) -> (86.5283, -124.2729) construction
  line L268 (100.7523, -91.2179) -> (114.7573, -91.2179)
  line L269 (114.7573, -91.2179) -> (114.7573, -105.2229)
  line L270 (114.7573, -105.2229) -> (100.7523, -105.2229)
  line L271 (100.7523, -105.2229) -> (100.7523, -91.2179)
  line L272 (100.7523, -91.2179) -> (114.7573, -105.2229) construction
  line L273 (114.7573, -91.2179) -> (100.7523, -105.2229) construction
  line L274 (105.5783, -110.2679) -> (119.5833, -110.2679)
  line L275 (119.5833, -110.2679) -> (119.5833, -124.2729)
  line L276 (119.5833, -124.2729) -> (105.5783, -124.2729)
  line L277 (105.5783, -124.2729) -> (105.5783, -110.2679)
  line L278 (105.5783, -110.2679) -> (119.5833, -124.2729) construction
  line L279 (119.5833, -110.2679) -> (105.5783, -124.2729) construction
  line L280 (96.1803, -129.3179) -> (110.1853, -129.3179)
  line L281 (110.1853, -129.3179) -> (110.1853, -143.3229)
  line L282 (110.1853, -143.3229) -> (96.1803, -143.3229)
  line L283 (96.1803, -143.3229) -> (96.1803, -129.3179)
  line L284 (96.1803, -129.3179) -> (110.1853, -143.3229) construction
  line L285 (110.1853, -129.3179) -> (96.1803, -143.3229) construction
  line L286 (115.2303, -129.3179) -> (129.2353, -129.3179)
  line L287 (129.2353, -129.3179) -> (129.2353, -143.3229)
  line L288 (129.2353, -143.3229) -> (115.2303, -143.3229)
  line L289 (115.2303, -143.3229) -> (115.2303, -129.3179)
  line L290 (115.2303, -129.3179) -> (129.2353, -143.3229) construction
  line L291 (129.2353, -129.3179) -> (115.2303, -143.3229) construction
  line L292 (124.6283, -110.2679) -> (138.6333, -110.2679)
  line L293 (138.6333, -110.2679) -> (138.6333, -124.2729)
  line L294 (138.6333, -124.2729) -> (124.6283, -124.2729)
  line L295 (124.6283, -124.2729) -> (124.6283, -110.2679)
  line L296 (124.6283, -110.2679) -> (138.6333, -124.2729) construction
  line L297 (138.6333, -110.2679) -> (124.6283, -124.2729) construction
  line L298 (119.8023, -91.2179) -> (133.8073, -91.2179)
  line L299 (133.8073, -91.2179) -> (133.8073, -105.2229)
  line L300 (133.8073, -105.2229) -> (119.8023, -105.2229)
  line L301 (119.8023, -105.2229) -> (119.8023, -91.2179)
  line L302 (119.8023, -91.2179) -> (133.8073, -105.2229) construction
  line L303 (133.8073, -91.2179) -> (119.8023, -105.2229) construction
  line L304 (138.8523, -91.2179) -> (152.8573, -91.2179)
  line L305 (152.8573, -91.2179) -> (152.8573, -105.2229)
  line L306 (152.8573, -105.2229) -> (138.8523, -105.2229)
  line L307 (138.8523, -105.2229) -> (138.8523, -91.2179)
  line L308 (138.8523, -91.2179) -> (152.8573, -105.2229) construction
  line L309 (152.8573, -91.2179) -> (138.8523, -105.2229) construction
  line L310 (143.6783, -110.2679) -> (157.6833, -110.2679)
  line L311 (157.6833, -110.2679) -> (157.6833, -124.2729)
  line L312 (157.6833, -124.2729) -> (143.6783, -124.2729)
  line L313 (143.6783, -124.2729) -> (143.6783, -110.2679)
  line L314 (143.6783, -110.2679) -> (157.6833, -124.2729) construction
  line L315 (157.6833, -110.2679) -> (143.6783, -124.2729) construction
  line L316 (134.2803, -129.3179) -> (148.2853, -129.3179)
  line L317 (148.2853, -129.3179) -> (148.2853, -143.3229)
  line L318 (148.2853, -143.3229) -> (134.2803, -143.3229)
  line L319 (134.2803, -143.3229) -> (134.2803, -129.3179)
  line L320 (134.2803, -129.3179) -> (148.2853, -143.3229) construction
  line L321 (148.2853, -129.3179) -> (134.2803, -143.3229) construction
  line L322 (153.3303, -129.3179) -> (167.3353, -129.3179)
  line L323 (167.3353, -129.3179) -> (167.3353, -143.3229)
  line L324 (167.3353, -143.3229) -> (153.3303, -143.3229)
  line L325 (153.3303, -143.3229) -> (153.3303, -129.3179)
  line L326 (153.3303, -129.3179) -> (167.3353, -143.3229) construction
  line L327 (167.3353, -129.3179) -> (153.3303, -143.3229) construction
  line L328 (157.9023, -91.2967) -> (171.9073, -91.2967)
  line L329 (171.9073, -91.2967) -> (171.9073, -105.3017)
  line L330 (171.9073, -105.3017) -> (157.9023, -105.3017)
  line L331 (157.9023, -105.3017) -> (157.9023, -91.2967)
  line L332 (157.9023, -91.2967) -> (171.9073, -105.3017) construction
  line L333 (171.9073, -91.2967) -> (157.9023, -105.3017) construction
  line L334 (162.7283, -110.2679) -> (176.7333, -110.2679)
  line L335 (176.7333, -110.2679) -> (176.7333, -124.2729)
  line L336 (176.7333, -124.2729) -> (162.7283, -124.2729)
  line L337 (162.7283, -124.2729) -> (162.7283, -110.2679)
  line L338 (162.7283, -110.2679) -> (176.7333, -124.2729) construction
  line L339 (176.7333, -110.2679) -> (162.7283, -124.2729) construction
  line L340 (176.9523, -91.2179) -> (190.9573, -91.2179)
  line L341 (190.9573, -91.2179) -> (190.9573, -105.2229)
  line L342 (190.9573, -105.2229) -> (176.9523, -105.2229)
  line L343 (176.9523, -105.2229) -> (176.9523, -91.2179)
  line L344 (176.9523, -91.2179) -> (190.9573, -105.2229) construction
  line L345 (190.9573, -91.2179) -> (176.9523, -105.2229) construction
  line L346 (181.7783, -110.2679) -> (195.7833, -110.2679)
  line L347 (195.7833, -110.2679) -> (195.7833, -124.2729)
  line L348 (195.7833, -124.2729) -> (181.7783, -124.2729)
  line L349 (181.7783, -124.2729) -> (181.7783, -110.2679)
  line L350 (181.7783, -110.2679) -> (195.7833, -124.2729) construction
  line L351 (195.7833, -110.2679) -> (181.7783, -124.2729) construction
  line L352 (172.3803, -129.3179) -> (186.3853, -129.3179)